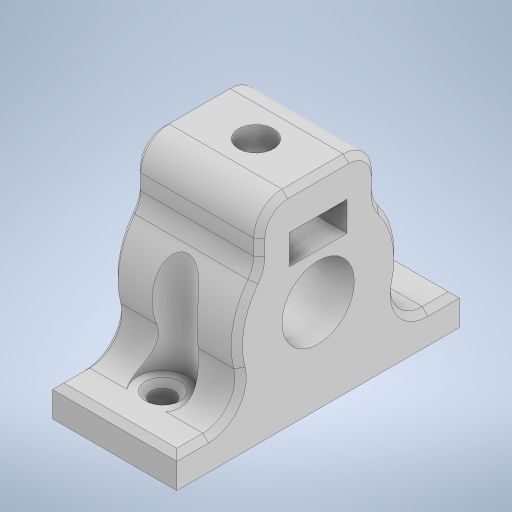
# Autodesk Inventor part: narishige_holder
Saved by Autodesk Inventor 2024 (Build 280153000, 153)
## iProperties
Created: 2021-05-18
Part Number: narishige_holder
Material: Generic
Document SubType Name: Modeling
Designer: Daniel
Density: 1 g/cm^3
Appearance: Default
Author: Daniel
Autodesk Inventor part; units mm, degrees
ref_plane "YZ Plane" through (0, 0, 0) normal (1, 0, 0) x (0, 1, 0)
sketch "Sketch1" plane through (0, 0, 0) normal (0, 1, 0) x (-1, 0, 0)
  line L0 (0, 0) -> (22, 0)
  line L1 (22, 0) -> (22, -50)
  line L2 (22, -50) -> (0, -50)
  line L3 (0, -50) -> (0, 0)
  circle A0 centre (11, -8.5) radius 2.05
  circle A1 centre (11, -41.5) radius 2.05
  line L4 (22, 0) -> (0, -50) construction
  line L5 (22, -50) -> (0, 0) construction
  point P0 (11, -25)
  dimension "d0" = 22
  dimension "d1" = 50
  dimension "d2" = 4.1
  dimension "d3" = 4.1
  dimension "d5" = 33
  dimension "d40" = 16.5
  constraints: 12 end point, 2 centre point, 2 parallel, 1 horizontal, 1 midpoint, 1 perpendicular, 1 vertical alignment
  measures "d0" distance of L1.end L2.end
  measures "d1" distance of L0.end L1.end
  measures "d2" diameter of A0
  measures "d3" diameter of A1
  measures "d5" distance of A0.centre A1.centre
  measures "d40" distance of point (11, -25) A0.centre
extrude "Extrusion1" add sketch "Sketch1" along normal blind 5.5
sketch "Sketch3" plane through (0, 0, 0) normal (1, 0, 0) x (0, 0, -1)
  circle A0 centre (25, 16.3589) radius 6.4
  circle A1 centre (25, 16.3589) radius 14.4
  line L0 (50, 5.5) -> (0, 5.5) projected
  arc A2 (5.6002, 5.5) -> (11.0873, 12.6443) centre (5.6002, 11.1793) ccw
  arc A3 (38.9127, 12.6443) -> (44.3998, 5.5) centre (44.3998, 11.1793) ccw
  line L1 (0, 5.5) -> (50, 5.5) projected
  point P0 (0, 0)
  point P1 (25, 5.5)
  dimension "d11" = 12.8
  dimension "d12" = 8
  constraints: 6 point on circle, 4 centre point, 4 tangent, 2 point on line, 1 coincident, 1 equal radius, 1 midpoint, 1 vertical alignment
  measures "d11" diameter of A0
  measures "d12" radial gap between concentric circles of A0 A1
extrude "Extrusion2" add sketch "Sketch3" against normal up to surface (22 mm away) contours A1 L0 | A1 L0 A2 | A3 L0 A1 picked at (24.7429, 7.0019)
sketch "Sketch4" plane through (0, 5.5, 0) normal (0, 1, 0) x (1, 0, 0)
  circle A0 centre (-11, 8.5) radius 2.05 construction
  circle A1 centre (-11, 8.5) radius 4.5
  circle A2 centre (-11, 41.5) radius 2.05 construction
  circle A3 centre (-11, 41.5) radius 4.5
  point P0 (0, 0)
  dimension "d15" = 9
  dimension "d16" = 9
  constraints: 2 centre point, 2 coincident
  measures "d15" diameter of A1
  measures "d16" diameter of A3
extrude "Extrusion3" cut sketch "Sketch4" along normal through all
ref_plane "Work Plane2" through (-11, 0, 0) normal (1, 0, 0) x (0, 0, -1)
sketch "Sketch11" plane through (0, 0, 0) normal (1, 0, 0) x (0, 0, -1)
  line L0 (14.5852, 24.3188) -> (35.4148, 24.3188)
  line L1 (35.4148, 24.3188) -> (35.4148, 30.915)
  line L2 (30.4148, 35.915) -> (19.5852, 35.915)
  line L3 (14.5852, 30.915) -> (14.5852, 24.3188)
  line L4 (0, 0) -> (50, 0) projected
  arc A0 (19.5852, 35.915) -> (14.5852, 30.915) centre (19.5852, 30.915) ccw
  arc A1 (35.4148, 30.915) -> (30.4148, 35.915) centre (30.4148, 30.915) ccw
  point P0 (35.4148, 35.915)
  point P1 (14.5852, 35.915)
  point P2 (25, 24.3188)
  point P3 (25, 0)
  dimension "d49" = 5
  constraints: 8 end point, 4 point on circle, 4 point on line, 4 tangent, 2 centre point, 2 midpoint, 2 parallel, 1 equal radius, 1 horizontal, 1 perpendicular, 1 vertical alignment
  measures "d49" radius of A0
extrude "Extrusion7" add sketch "Sketch11" against normal up to surface (22 mm away)
sketch "Sketch7" plane through (-11, 0, 0) normal (1, 0, 0) x (0, 0, -1)
  arc A0 (38.9127, 12.6443) -> (11.0873, 12.6443) centre (25, 16.3589) ccw construction
  line L0 (25, 16.3589) -> (25, 53.8517)
  line L1 (25, 40.4327) -> (28.1, 40.4327)
  line L2 (28.1, 40.4327) -> (28.1, 27.8589)
  line L3 (28.1, 27.8589) -> (28.1, 21.958)
  line L4 (28.1, 21.958) -> (25, 21.958)
  circle A1 centre (25, 16.3589) radius 6.4 projected
  point P0 (0, 0)
  point P1 (25, 22.7589)
  point P2 (28.1, 30.4212)
  point P3 (25, 30.7589)
  dimension "d28" = 6.2
  constraints: 10 end point, 3 point on line, 2 collinear, 2 perpendicular, 2 point on circle, 1 horizontal, 1 vertical
  measures "d28" diameter of L2 L0
revolve "Revolution1" cut sketch "Sketch7" angle 360 about axis through (-11, 16.3589, -25) along (0, 1, 0) picked at (26.7389, 22.1049) contours L0 A1 L4 | L0 L1 L2 L3 A1
ref_plane "Work Plane3" through (0, 27, 0) normal (0, -1, 0) x (1, 0, 0)
sketch "Sketch10" plane through (0, 27, 0) normal (0, -1, 0) x (1, 0, 0)
  line L0 (-16.889, -25) -> (-13.9445, -19.9)
  line L1 (-13.9445, -19.9) -> (-8.0555, -19.9)
  line L2 (-8.0555, -19.9) -> (-5.111, -25) construction
  line L3 (-5.111, -25) -> (-8.0555, -30.1) construction
  line L4 (-8.0555, -30.1) -> (-13.9445, -30.1)
  line L5 (-13.9445, -30.1) -> (-16.889, -25)
  line L6 (-8.0555, -19.9) -> (0, -19.9)
  line L7 (0, -19.9) -> (0, -30.1)
  line L8 (0, -30.1) -> (-8.0555, -30.1)
  circle A0 centre (-11, -25) radius 3.1 projected
  point P0 (0, 0)
  point P1 (-11, -21.9)
  dimension "d44" = 10.2
  constraints: 18 end point, 2 horizontal, 2 perpendicular, 1 coincident, 1 vertical alignment, 13 other
  measures "d44" distance between parallel lines of L4 L1
extrude "Extrusion6" cut sketch "Sketch10" along normal mid plane 5.2 contours L0 L1 L6 L7 L8 L4 L5 | A0
fillet "Fillet1" radius 5 2 edges at (-11, 26.3033, -35.4148) (-11, 26.3033, -14.5852)
chamfer "Chamfer1" distance 1 angle 45 22 edges at (-11, 5.5, 0) (-11, 5.5, -50) (0, 7.72, -10.1044) (0, 5.5, -2.8001) (0, 19.1603, -10.8751) (0, 19.1603, -39.1249) (0, 7.72, -39.8956) (0, 5.5, -47.1999) (-22, 19.1603, -39.1249) (-22, 7.72, -39.8956) (-22, 5.5, -47.1999) (-22, 19.1603, -10.8751) (-22, 7.72, -10.1044) (-22, 5.5, -2.8001) (-8.95, 5.5, -8.5) (-8.95, 5.5, -41.5) (0, 29.5264, -14.5852) (0, 29.5264, -35.4148) (0, 35.915, -25) (-22, 29.5264, -35.4148) (-22, 29.5264, -14.5852) (-22, 35.915, -25)
body "Solid1"
